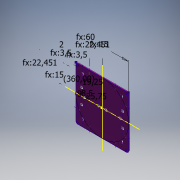
# Autodesk Inventor part: pcb_board
Saved by Autodesk Inventor 2019 (Build 230136000, 136)
## iProperties
Created: 2018-04-27
Part Number: pcb_board
Material: ABS Plastic
Document SubType Name: Modeling
Designer: Fierl
Density: 1.06 g/cm^3
Appearance: Smooth - White
Mass: 5.5583 g
Surface Area: 75.5753 cm^2
Volume: 5.24368 cm^3
Author: Fierl
Autodesk Inventor part; units mm, degrees
ref_plane "YZ Plane" through (0, 0, 0) normal (1, 0, 0) x (0, 1, 0)
ref_plane "XZ Plane" through (0, 0, 0) normal (0, 1, 0) x (-1, 0, 0)
ref_plane "XY Plane" through (0, 0, 0) normal (0, 0, 1) x (1, 0, 0)
sketch "Sketch1" plane through (0, 0, 0) normal (0, 0, 1) x (1, 0, 0)
  line L0 (0, -42.5799) -> (0, 42.5799) projected
  line L1 (-42.5799, 0) -> (42.5799, 0) projected
  line L2 (-28, 30) -> (28, 30)
  line L3 (30, 28) -> (30, -28)
  line L4 (28, -30) -> (-28, -30)
  line L5 (-30, -28) -> (-30, 28)
  arc A0 (-28, 30) -> (-30, 28) centre (-28, 28) ccw
  arc A1 (30, 28) -> (28, 30) centre (28, 28) ccw
  arc A2 (28, -30) -> (30, -28) centre (28, -28) ccw
  arc A3 (-30, -28) -> (-28, -30) centre (-28, -28) ccw
  point P0 (0, 0)
  point P1 (-30, 30)
  point P2 (30, 30)
  point P3 (-22.4506, 22.4506)
  point P4 (-26.5, 15)
  point P5 (-15, 26.5)
  point P6 (-15, -26.5)
  point P7 (-22.4506, -22.4506)
  point P8 (-26.5, -15)
  point P9 (26.5, -15)
  point P10 (22.4506, -22.4506)
  point P11 (15, -26.5)
  point P12 (15, 26.5)
  point P13 (22.4506, 22.4506)
  point P14 (26.5, 15)
  point P15 (-21, 0)
  point P16 (21, 0)
  point P17 (-4.25, 0)
  point P18 (4.25, 0)
  point P19 (-23.5, 8.5)
  point P20 (-23.5, -8.5)
  point P21 (23.5, 8.5)
  point P22 (23.5, -8.5)
  dimension "d0" = 60
  dimension "d1" = 2
  dimension "d2" = 22.4506
  dimension "d3" = 22.4506
  dimension "d4" = 15
  dimension "d5" = 15
  dimension "d6" = 3.5
  dimension "d7" = 3.5
  dimension "d10" = 360
  dimension "d28" = 9
  dimension "d36" = 25.75
  dimension "d48" = 19.25
  dimension "d49" = 8.5
  constraints: 8 end point, 8 point on circle, 8 tangent, 7 point on line, 5 symmetric about line, 4 centre point, 3 equal radius, 2 parallel, 2 perpendicular, 1 horizontal, 15 other
  measures "d0" distance of point (-30, 30) point (30, 30)
  measures "d1" radius of A0
  measures "d2" distance from line of L0 point (-22.451, 22.451)
  measures "d3" distance from line of L1 point (-22.451, 22.451)
  measures "d4" distance from line of L1 point (-26.5, 15)
  measures "d5" distance from line of L0 point (-15, 26.5)
  measures "d6" distance from line of L2 point (-15, 26.5)
  measures "d7" distance from line of L5 point (-26.5, 15)
  measures "d28" distance from line of L5 point (-21, 0)
  measures "d36" distance from line of L5 point (-4.25, 0)
  measures "d48" horizontal distance of point (-4.25, 0) point (-23.5, 8.5)
  measures "d49" distance from line of L1 point (-23.5, 8.5)
extrude "Extrusion1" add sketch "Sketch1" against normal blind 1.5
hole "Hole1" at (-22.4506, 22.4506, 0) at (22.4506, 22.4506, 0) at (22.4506, -22.4506, 0) at (-22.4506, -22.4506, 0) direction (0, 0, -1) diameter 3.4 end through all clearance for "Countersunk Flat Head Screw DIN EN ISO 2009" size "M3" standard "DIN"
hole "Hole2" at (-26.5, 15, 0) at (-15, 26.5, 0) at (-15, -26.5, 0) at (-26.5, -15, 0) at (26.5, -15, 0) at (15, -26.5, 0) at (15, 26.5, 0) at (26.5, 15, 0) direction (0, 0, -1) diameter 2.4 end through all clearance for "Countersunk Flat Head Screw DIN EN ISO 2009" size "M2" standard "DIN"
hole "Hole3" at (-21, 0, 0) at (21, 0, 0) direction (0, 0, -1) diameter 3 end through all
hole "Hole4" at (-4.25, 0, 0) at (4.25, 0, 0) at (-23.5, -8.5, 0) at (-23.5, 8.5, 0) at (23.5, 8.5, 0) at (23.5, -8.5, 0) direction (0, 0, -1) diameter 3 end through all
equation "\"d0\" = backplate_width"
equation "\"d2\" = hole_distance"
equation "\"d3\" = hole_distance"
equation "\"d4\" = screw_distance_center"
equation "\"d5\" = screw_distance_center"
equation "\"d6\" = screw_distance_outside"
equation "\"d7\" = screw_distance_outside"
equation "\"encoder_axis\" = 8"
equation "\"encoder_emboss\" = 0"
equation "\"encoders\" = 0"
equation "\"encoder_width\" = 27"
equation "\"front_plate_thickness\" = 2"
equation "\"glass_thickness\" = 2"
equation "\"screw_distance_outside\" = 3.5"
equation "\"encoder_rad\" = 49"
equation "\"encoder_extrude_hight\" = 3"
equation "\"screw_distance_center\" = 15"
equation "\"ring_top_thickness\" = 2"
equation "\"ring_outer_bevel_depth\" = 0.5"
equation "\"ring_depth\" = 6"
equation "\"ring_outer_bevel_height\" = 3"
equation "\"ring_inner_bevel_depth\" = 3.5"
equation "\"ring_thickness\" = 9"
equation "\"hole_from_center\" = 63.5"
equation "\"circle_dimension_inner\" = 47"
equation "\"circle_dimension\" = 56"
equation "\"backplate_width\" = 60"
equation "\"hole_distance\" = 22.45064"
body "Solid1"
